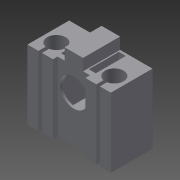
# Autodesk Inventor part: XCarriageV5
Saved by Autodesk Inventor 2015 (Build 190159000, 159)
## iProperties
Created: 2014-08-18
Part Number: XCarriageV5
Material: Generic
Document SubType Name: Modeling
Designer: Jack
Density: 1 g/cm^3
Appearance: Default
Author: Jack
Autodesk Inventor part; units mm, degrees
ref_plane "YZ Plane" through (0, 0, 0) normal (1, 0, 0) x (0, 1, 0)
ref_plane "XZ Plane" through (0, 0, 0) normal (0, 1, 0) x (-1, 0, 0)
ref_plane "XY Plane" through (0, 0, 0) normal (0, 0, 1) x (1, 0, 0)
sketch "Sketch1" plane through (0, 0, 0) normal (0, 0, 1) x (1, 0, 0)
  arc A0 (1.5, -7.8581) -> (-1.5, -7.8581) centre (0, 0) ccw
  arc A1 (51.5, -7.8581) -> (48.5, -7.8581) centre (50, 0) ccw
  line L0 (-11, -14) -> (-11, 22)
  line L1 (-11, 22) -> (61, 22)
  line L2 (61, 22) -> (61, -14)
  line L3 (39, -14) -> (39, -10)
  line L4 (39, -10) -> (11, -10)
  line L5 (11, -10) -> (11, -14)
  line L6 (51.5, -14) -> (51.5, -7.8581)
  line L7 (48.5, -14) -> (48.5, -7.8581)
  line L8 (1.5, -7.8581) -> (1.5, -14)
  line L9 (-1.5, -7.8581) -> (-1.5, -14)
  line L10 (61, -14) -> (51.5, -14)
  line L11 (48.5, -14) -> (39, -14)
  line L12 (11, -14) -> (1.5, -14)
  line L13 (-1.5, -14) -> (-11, -14)
  dimension "d0" = 16
  dimension "d1" = 16
  dimension "d2" = 50
  dimension "d3" = 22
  dimension "d4" = 10
  dimension "d6" = 11
  dimension "d7" = 11
  dimension "d8" = 11
  dimension "d9" = 11
  dimension "d14" = 1.5
  dimension "d15" = 1.5
  dimension "d16" = 1.5
  dimension "d17" = 1.5
  dimension "d18" = 14
  constraints: 28 end point, 12 perpendicular, 4 horizontal alignment, 4 point on circle, 4 vertical, 2 centre point, 1 coincident
  measures "d0" diameter of A0
  measures "d1" diameter of A1
  measures "d2" distance of A1.centre point (0, 0)
  measures "d3" distance from line of A1.centre L1
  measures "d4" distance from line of point (0, 0) L4
  measures "d6" distance from line of L0 point (0, 0)
  measures "d7" distance from line of L2 A1.centre
  measures "d8" distance from line of A1.centre L3
  measures "d9" distance from line of L5 point (0, 0)
  measures "d14" distance from line of A1.centre L7
  measures "d15" distance from line of A1.centre L6
  measures "d16" distance from line of point (0, 0) L9
  measures "d17" distance from line of point (0, 0) L8
  measures "d18" distance from line of A1.centre L11
extrude "Extrusion1" add sketch "Sketch1" along normal blind 60
sketch "Sketch2" plane through (11, -10, 0) normal (0, -1, 0) x (1, 0, 0)
  line L0 (0, 60) -> (28, 60) projected
  circle A0 centre (14, 40) radius 12
  line L1 (28, 0) -> (28, 60) projected
  line L2 (50, 0) -> (50, 60) projected
  point P0 (-11, 0)
  dimension "d12" = 24
  dimension "d13" = 20
  dimension "d24" = 36
  constraints: 1 centre point
  measures "d12" diameter of A0
  measures "d13" distance from line of L0 A0.centre
  measures "d24" distance from line of L2 A0.centre
extrude "Extrusion2" cut sketch "Sketch2" against normal blind 26
sketch "Sketch3" plane through (25, 16, 40) normal (0, -1, 0) x (1, 0, 0)
  circle A0 centre (0, 0) radius 12 projected
  circle A1 centre (0, 0) radius 8
  point P0 (-25, -40)
  dimension "d21" = 16
  constraints: 1 centre point, 1 coincident
  measures "d21" diameter of A1
extrude "Extrusion3" cut sketch "Sketch3" against normal up to surface (6 mm away) contours A1
sketch "Sketch5" plane through (0, 0, 60) normal (0, 0, 1) x (1, 0, 0)
  line L0 (11, -14) -> (11, -10) projected
  line L1 (11, -10) -> (39, -10) projected
  line L2 (39, -10) -> (39, -14) projected
  line L3 (61, 22) -> (-11, 22) projected
  line L4 (17, -10) -> (33, -10)
  line L5 (33, -10) -> (33, 22)
  line L6 (33, 22) -> (17, 22)
  line L7 (17, 22) -> (17, -10)
  dimension "d31" = 6
  dimension "d32" = 6
  constraints: 8 end point, 2 parallel, 2 point on line, 1 horizontal, 1 perpendicular
  measures "d31" distance between parallel lines of L2 L5
  measures "d32" distance between parallel lines of L0 L7
extrude "Extrusion5" add sketch "Sketch5" along normal blind 10
ref_plane "Work Plane1" through (0, 0, 26) normal (0, 0, -1) x (-1, 0, 0)
sketch "Sketch6" plane through (0, 0, 26) normal (0, 0, -1) x (-1, 0, 0)
  line L0 (-17, 22) -> (11, 22) projected
  line L1 (-61, 22) -> (-33, 22) projected
  line L2 (-40, 22) -> (-10, 22)
  line L3 (-10, 22) -> (-10, -8)
  line L4 (-13, -10) -> (-37, -10) projected
  line L5 (-10, -8) -> (-40, -8)
  line L6 (-40, -8) -> (-40, -5.7247)
  line L7 (-40, -5.7247) -> (-40, 22)
  point P0 (0, 0)
  dimension "d36" = 30
  dimension "d37" = 21
  dimension "d38" = 30
  dimension "d39" = 30
  constraints: 10 end point, 2 point on line, 1 collinear, 1 horizontal, 1 perpendicular
  measures "d36" distance of L2.start L2.end
  measures "d37" distance of L0.end L2.end
  measures "d38" distance of L2.end L3.end
  measures "d39" distance of L3.end L5.end
extrude "Extrusion6" cut sketch "Sketch6" along normal blind 10 and the other way blind 13
sketch "Sketch7" plane through (0, 0, 60) normal (0, 0, 1) x (1, 0, 0)
  line L0 (33, 22) -> (33, -10) projected
  line L1 (17, -10) -> (17, 22) projected
  line L2 (17, 22) -> (-11, 22) projected
  line L3 (-11, 22) -> (-11, -14) projected
  line L4 (-11, -14) -> (-1.5, -14) projected
  line L5 (-1.5, -14) -> (-1.5, -7.8581) projected
  arc A0 (1.5, -7.8581) -> (-1.5, -7.8581) centre (0, 0) ccw projected
  line L6 (1.5, -7.8581) -> (1.5, -14) projected
  line L7 (1.5, -14) -> (11, -14) projected
  line L8 (11, -14) -> (11, -10) projected
  line L9 (11, -10) -> (17, -10) projected
  line L10 (16, 20) -> (10, 20)
  line L11 (10, 20) -> (10, -6)
  line L12 (10, -6) -> (16, -6)
  line L13 (16, -6) -> (16, 20)
  line L14 (34, 20) -> (40, 20)
  line L15 (40, 20) -> (40, -6)
  line L16 (40, -6) -> (34, -6)
  line L17 (34, -6) -> (34, 20)
  dimension "d44" = 6
  dimension "d45" = 6
  dimension "d46" = 1
  dimension "d47" = 1
  dimension "d48" = 26
  dimension "d49" = 26
  dimension "d50" = 2
  constraints: 16 end point, 4 parallel, 2 horizontal, 2 perpendicular, 1 point on line
  measures "d44" distance of L14.start L14.end
  measures "d45" distance of L10.start L10.end
  measures "d46" distance between parallel lines of L1 L13
  measures "d47" distance between parallel lines of L0 L17
  measures "d48" distance of L14.end L15.end
  measures "d49" distance of L10.end L11.end
  measures "d50" distance between parallel lines of L2 L10
extrude "Extrusion7" cut sketch "Sketch7" against normal blind 21.75 contours L13 L12 L11 L10 | L14 L15 L16 L17
body "Solid1"
